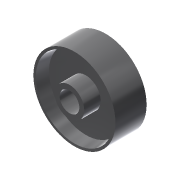
# Autodesk Inventor part: Wheel
Saved by Autodesk Inventor 2022 Beta2 (Build 260130000, 130) ContinuousBuild 0
## iProperties
Created: 2007-03-01
Part Number: Wheel
Document SubType Name: Modeling
Designer: MFlayler
Material: Thermoplastic Resin
Mass: 166.892 g
Surface Area: 420.538 cm^2
Volume: 130.384 cm^3
Density: 1.28 g/cm^3
Appearance: Smooth - Medium Gray
Author: MFlayler
Autodesk Inventor part; units mm, degrees
ref_plane "YZ Plane" through (0, 0, 0) normal (1, 0, 0) x (0, 1, 0)
ref_plane "XZ Plane" through (0, 0, 0) normal (0, 1, 0) x (-1, 0, 0)
ref_plane "XY Plane" through (0, 0, 0) normal (0, 0, 1) x (1, 0, 0)
sketch "Sketch1" plane through (0, 0, 0) normal (0, 0, 1) x (1, 0, 0)
  line L0 (0, 40) -> (0, -30) projected
  line L1 (8.2, 0) -> (61.4, 0) projected
  line L2 (12, 25) -> (12, -25)
  line L3 (12, 25) -> (18, 25)
  line L4 (18, 25) -> (18, 5)
  line L5 (18, 5) -> (45, 5)
  line L6 (47, 19) -> (50, 19)
  line L7 (50, 19) -> (50, -19)
  line L8 (50, -19) -> (47, -19)
  line L9 (47, -19) -> (45, -5)
  line L10 (45, -5) -> (18, -5)
  line L11 (18, -5) -> (18, -25)
  line L12 (18, -25) -> (12, -25)
  line L13 (45, 5) -> (47, 19)
  dimension "d0" = 50
  dimension "d1" = 24
  dimension "d2" = 36
  dimension "d3" = 100
  dimension "d4" = 3
  dimension "d5" = 10
  dimension "d6" = 5
  dimension "d7" = 38
  constraints: 24 end point, 6 parallel, 3 equal length, 3 perpendicular, 1 collinear, 3 other
  measures "d0" distance of L2.start L2.end
  measures "d1" diameter of L2 L0
  measures "d2" diameter of L4 L0
  measures "d3" diameter of L7 L0
  measures "d4" distance of L6.start L6.end
  measures "d5" distance between parallel lines of L10 L5
  measures "d6" distance from line of L7 L9.end
  measures "d7" distance of L6.end L7.end
revolve "Revolution1" add sketch "Sketch1" angle 360 about axis through (0, 0, 0) along (0, -1, 0)
body "Solid1"
